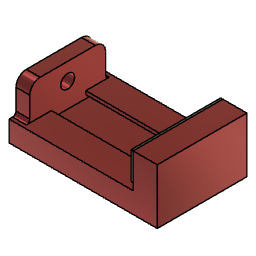
vise body v1 (Autodesk Fusion 360 design; units mm, degrees)
Autodesk Fusion 360 part; units mm, degrees
sketch "Sketch1" plane through (0, 0, 0) normal (0, 1, 0) x (1, 0, 0)
  line L0 (-85, 0) -> (95, 0)
  line L1 (95, 0) -> (95, -50)
  line L2 (95, -50) -> (130, -50)
  line L3 (130, -50) -> (130, 30)
  line L4 (130, 30) -> (-85, 30)
  line L5 (-85, 30) -> (-85, 0)
  dimension "d1" = 80
  dimension "d2" = 215
  dimension "d3" = 30
  dimension "d4" = 50
  dimension "d5" = 35
  constraint horizontal L0
  constraint perpendicular L0 L1
  constraint perpendicular L1 L2
  constraint perpendicular L2 L3
  constraint perpendicular L0 L5
  measures "d1" distance of L2 L3.end
  measures "d2" distance of L3.end L4.end
  measures "d3" distance of L0.start L4.end
  measures "d4" distance of L0.end L1.end
  measures "d5" distance of L1.end L2.end
extrude "Extrude1" add sketch "Sketch1" along normal blind 130 makes body 1
sketch "Sketch2" plane through (-85, 0, 0) normal (-1, 0, 0) x (0, -1, 0)
  line L0 (0, -30) -> (0, 0)
  line L1 (0, 0) -> (-130, 0)
  line L2 (-130, 0) -> (-130, -30)
  line L3 (-130, -30) -> (0, -30)
  line L4 (-120, 5) -> (-120, 35)
  line L5 (-105, 50) -> (-25, 50)
  line L6 (-10, 35) -> (-10, 5)
  line L7 (-130, 0) -> (-130, 50)
  line L8 (0, 0) -> (0, 50)
  arc A0 (-105, 50) -> (-120, 35) centre (-105, 35) ccw
  line L9 (-130, 0) -> (-125, 0)
  arc A1 (-125, 0) -> (-120, 5) centre (-125, 5) ccw
  arc A2 (-10, 35) -> (-25, 50) centre (-25, 35) ccw
  line L10 (0, 0) -> (-5, 0)
  arc A3 (-10, 5) -> (-5, 0) centre (-5, 5) ccw
  circle A4 centre (-65, 25) radius 10
  dimension "d8" = 10
  dimension "d9" = 10
  dimension "d10" = 15
  dimension "d11" = 5
  dimension "d12" = 15
  dimension "d13" = 5
  dimension "d14" = 20
  dimension "d15" = 25
  dimension "d16" = 65
  constraint perpendicular L1 L4
  constraint perpendicular L4 L5
  constraint perpendicular L1 L6
  constraint tangent L4 A0
  constraint tangent L5 A0
  constraint coincident L1.end L2.start
  constraint tangent L4 A1
  constraint tangent L9 A1
  constraint tangent L6 A2
  constraint tangent L5 A2
  constraint coincident L0.end L1.start
  constraint tangent L10 A3
  constraint tangent L6 A3
  measures "d8" distance of L4 L7
  measures "d9" distance of L6 L8
  measures "d10" radius of A0
  measures "d11" radius of A1
  measures "d12" radius of A2
  measures "d13" radius of A3
  measures "d14" diameter of A4
  measures "d15" distance of L5 A4.centre
  measures "d16" distance of L2 A4.centre
extrude "Extrude2" add sketch "Sketch2" against normal blind 20 contours L1 L4 L5 L6 A0 A1 A2 A3 bodies 1
sketch "Sketch3" plane through (0, 0, 0) normal (1, 0, 0) x (0, 1, 0)
  line L0 (130, 0) -> (0, 0)
  line L1 (66.3285, 25) -> (66.3285, -32.6161) construction
  line L2 (41.3285, -5) -> (26.3285, -10)
  line L3 (26.3285, -10) -> (66.3285, -10)
  line L4 (41.3285, -5) -> (41.3285, 0)
  line L5 (91.3285, -5) -> (91.3285, 0)
  line L6 (91.3285, -5) -> (106.3285, -10)
  line L7 (106.3285, -10) -> (66.3285, -10)
  line L8 (41.3285, 0) -> (91.3285, 0)
  dimension "d19" = 5
  dimension "d20" = 40
  dimension "d21" = 25
  dimension "d26" = 130
  dimension "d27" = 10
  constraint coincident L0.end origin
  constraint horizontal L0
  constraint vertical L1
  constraint coincident L0 L4.end
  constraint coincident L1 L3.end
  constraint perpendicular L1 L3
  constraint symmetric L1 L4.end L5.end
  constraint symmetric L1 L2.start L5.start
  constraint symmetric L1 L2.end L6.end
  constraint symmetric L1 L3.end L7.end
  measures "d19" distance of L4.end L2.start
  measures "d20" distance of L2.end L3.end
  measures "d21" distance of L1 L4
  measures "d26" distance of L0.start L0.end
  measures "d27" distance of L3 L8
extrude "Extrude3" cut sketch "Sketch3" along normal blind 95 and the other way blind 65 bodies 1
sketch "Sketch4" plane through (95, 0, 0) normal (-1, 0, 0) x (0, -1, 0)
  line L0 (0, 0) -> (0, 50)
  line L1 (0, 50) -> (-130, 50)
  line L2 (-130, 50) -> (-130, 0)
  line L3 (-130, 0) -> (-91.3285, 0)
  line L4 (-91.3285, 0) -> (-91.3285, -5)
  line L5 (-91.3285, -5) -> (-106.3285, -10)
  line L6 (-106.3285, -10) -> (-26.3285, -10)
  line L7 (-26.3285, -10) -> (-41.3285, -5)
  line L8 (-41.3285, -5) -> (-41.3285, 0)
  line L9 (-41.3285, 0) -> (0, 0)
  line L10 (-130, 50) -> (0, 50)
  line L11 (0, 10) -> (0, 50)
  line L12 (-130, 50) -> (-130, 10)
  line L13 (-130, 10) -> (0, 10)
  dimension "d28" = 40
  constraint coincident L1.end L2.start
  constraint coincident L0.end L1.start
  constraint coincident L0 L11.start
  constraint perpendicular L10 L11
  constraint coincident L2 L12.end
  constraint perpendicular L10 L12
  measures "d28" distance of L1.end L12.end
extrude "Extrude4" add sketch "Sketch4" along normal blind 3 separate body contours L0 L1 L2 L10 L11 L12 L13 makes body 2
